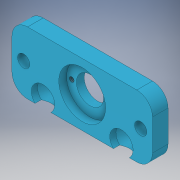
# Autodesk Inventor part: CHA_010_EncoderMountRev0
Saved by Autodesk Inventor 2018.3 (Build 223284000, 284)
## iProperties
Created: 2017-01-19
Part Number: CHA_010_EncoderMountRev0
Material: ABS Plastic
Document SubType Name: Modeling
Designer: xieedwa
Density: 1.06 g/cm^3
Appearance: Turquoise
Mass: 8.37617 g
Surface Area: 40.3255 cm^2
Volume: 7.90205 cm^3
Author: xieedwa
Autodesk Inventor part; units mm, degrees
ref_plane "YZ Plane" through (0, 0, 0) normal (1, 0, 0) x (0, 1, 0)
ref_plane "XZ Plane" through (0, 0, 0) normal (0, 1, 0) x (-1, 0, 0)
ref_plane "XY Plane" through (0, 0, 0) normal (0, 0, 1) x (1, 0, 0)
sketch "Sketch1" plane through (0, 0, 0) normal (0, 0, 1) x (1, 0, 0)
  line L0 (-28.575, -12.7) -> (28.575, -12.7)
  line L1 (28.575, -12.7) -> (28.575, 12.7)
  line L2 (28.575, 12.7) -> (-28.575, 12.7)
  line L3 (-28.575, 12.7) -> (-28.575, -12.7)
  point P0 (0, 0)
  dimension "d0" = 57.15
  dimension "d1" = 25.4
  dimension "d33" = 28.575
  dimension "d34" = 12.7
  constraints: 8 end point, 2 parallel, 1 horizontal, 1 perpendicular, 1 other
  measures "d0" distance of L1.end L2.end
  measures "d1" distance of L2.end L0.start
  measures "d33" distance from line of point (0, 0) L3
  measures "d34" distance from line of L0 point (0, 0)
extrude "Extrusion1" add sketch "Sketch1" along normal blind 3.175 and the other way blind 3.175
sketch "Sketch2" plane through (0, 0, 3.175) normal (0, 0, 1) x (1, 0, 0)
  line L0 (-28.575, -12.7) -> (28.575, -12.7) projected
  line L1 (28.575, -12.7) -> (28.575, 12.7) projected
  line L2 (28.575, 12.7) -> (-28.575, 12.7) projected
  line L3 (-28.575, 12.7) -> (-28.575, -12.7) projected
  point P0 (0, 0)
  point P1 (0, 0)
  dimension "d4" = 28.575
  dimension "d5" = 12.7
  dimension "d6" = 57.15
  measures "d4" distance from line of L1 point (0, 0)
  measures "d5" distance from line of L2 point (0, 0)
  measures "d6" distance of L1.end L2.end
hole "Hole1" at (0, 0, 3.175) direction (0, 0, -1) diameter 11.1125 end through all counterbore diameter 19.05 counterbore depth 3.175
sketch "Sketch3" plane through (0, 0, 3.175) normal (0, 0, 1) x (1, 0, 0)
  circle A0 centre (0, 0) radius 9.525 projected
  line L0 (-28.575, -12.7) -> (28.575, -12.7) projected
  line L1 (28.575, -12.7) -> (28.575, 12.7) projected
  line L2 (28.575, 12.7) -> (-28.575, 12.7) projected
  line L3 (-28.575, 12.7) -> (-28.575, -12.7) projected
  point P0 (0, 0)
  point P1 (-23.8124, -0.0762)
  point P2 (23.8124, -0.0762)
  dimension "d14" = 23.8125
  dimension "d15" = 23.8125
  dimension "d59" = 0.0762
  constraints: 1 horizontal alignment
  measures "d14" distance of point (-23.812, -0.076) A0.centre
  measures "d15" distance of A0.centre point (23.812, -0.076)
  measures "d59" vertical distance of point (0, 0) point (-23.812, -0.076)
hole "Hole2" at (-23.8124, -0.0762, 3.175) at (23.8124, -0.0762, 3.175) direction (0, 0, -1) diameter 4.9784 end through all clearance for "Flat Head Machine Screw (82)" size "#10" standard "Ansi Unified Screw Threads"
sketch "Sketch4" plane through (0, 0, 3.175) normal (0, 0, 1) x (1, 0, 0)
  circle A0 centre (-23.8124, -0.0762) radius 2.4892 projected
  circle A1 centre (23.8124, -0.0762) radius 2.4892 projected
  circle A2 centre (0, 0) radius 9.525 projected
  line L0 (-28.575, -12.7) -> (28.575, -12.7) projected
  line L1 (28.575, -12.7) -> (28.575, 12.7) projected
  line L2 (28.575, 12.7) -> (-28.575, 12.7) projected
  line L3 (-28.575, 12.7) -> (-28.575, -12.7) projected
  point P0 (0, 0)
  point P1 (-7.4422, 0)
  point P2 (7.4422, 0)
  dimension "d23" = 7.4422
  dimension "d24" = 7.4422
  constraints: 2 horizontal alignment
  measures "d23" distance of A2.centre point (-7.442, 0)
  measures "d24" distance of A2.centre point (7.442, 0)
hole "Hole3" at (-7.4422, 0, 3.175) at (7.4422, 0, 3.175) direction (0, 0, -1) diameter 1.9304 end through all
fillet "Fillet1" radius 6.35 4 edges at (28.575, 12.7, 0) (-28.575, 12.7, 0) (-28.575, -12.7, 0) (28.575, -12.7, 0)
sketch "Sketch5" plane through (0, 0, 3.175) normal (0, 0, 1) x (1, 0, 0)
  line L0 (28.575, -6.35) -> (28.575, 6.35) projected
  line L1 (-28.575, 6.35) -> (-28.575, -6.35) projected
  line L2 (-22.225, -12.7) -> (22.225, -12.7) projected
  line L3 (22.225, 12.7) -> (-22.225, 12.7) projected
  point P0 (0, 0)
  point P1 (15.9512, -9.1948)
  point P2 (-15.9512, -9.1948)
  dimension "d41" = 12.6238
  dimension "d42" = 12.6238
  dimension "d43" = 3.5052
  constraints: 1 horizontal alignment
  measures "d41" distance from line of L0 point (15.951, -9.195)
  measures "d42" distance from line of L1 point (-15.951, -9.195)
  measures "d43" distance from line of L2 point (-15.951, -9.195)
hole "Hole5" at (15.9512, -9.1948, 3.175) at (-15.9512, -9.1948, 3.175) direction (0, 0, -1) diameter 9.525 depth 2.54 tip angle 118
equation "\"d33\" = 0.5 * d0"
equation "\"d34\" = 0.5 * d1"
equation "\"d4\" = 0.5 * d6"
equation "\"d15\" = d14"
equation "\"d24\" = d23"
body "Solid1"
